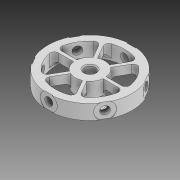
# Autodesk Inventor part: DrivePulley
Saved by Autodesk Inventor 2020 (Build 240168000, 168)
## iProperties
Created: 2021-05-16
Part Number: DrivePulley
Material: Generic
Document SubType Name: Modeling
Designer: DDeGo
Density: 1 g/cm^3
Appearance: Default
Author: DDeGo
Autodesk Inventor part; units mm, degrees
ref_plane "YZ Plane" through (0, 0, 0) normal (1, 0, 0) x (0, 1, 0)
ref_plane "XZ Plane" through (0, 0, 0) normal (0, 1, 0) x (-1, 0, 0)
sketch "Sketch1" plane through (0, 0, 0) normal (0, 0, 1) x (1, 0, 0)
  line L0 (5.5, 9.1) -> (5.5, 7.6)
  line L1 (5.5, 7.6) -> (4, 7.1)
  line L2 (4, 7.1) -> (4, 3.5)
  line L3 (4, 3.5) -> (5.5, 3)
  line L4 (5.5, 3) -> (5.5, 0)
  line L5 (5.5, 0) -> (2.57, 0)
  line L6 (2.57, 0) -> (2.57, 9.1)
  line L7 (2.57, 9.1) -> (5.5, 9.1)
  line L8 (2.57, 0) -> (0, 0) construction
  line L9 (0, 0) -> (0, 9.1) construction
  line L10 (0, 9.1) -> (2.57, 9.1) construction
  dimension "d1" = 3.6
  dimension "d2" = 1.5
  dimension "d3" = 3
  dimension "d4" = 0.5
  dimension "d5" = 1.5
  dimension "d15" = 2.57
  dimension "d16" = 4
  constraints: 22 end point, 4 perpendicular, 2 point on line, 1 equal length, 1 horizontal, 1 parallel, 1 vertical, 1 other
  measures "d1" distance of L2.start L3.start
  measures "d2" distance of L0.start L1.start
  measures "d3" distance of L4.start L4.end
  measures "d4" vertical distance of L3.start L4.start
  measures "d5" distance between parallel lines of L2 L4
  measures "d15" distance between parallel lines of L6 L9
  measures "d16" distance between parallel lines of L9 L2
revolve "Revolution1" add sketch "Sketch1" angle 360 about axis through (0, 0, 0) along (0, 1, 0)
sketch "Sketch2" plane through (0, 0, 0) normal (1, 0, 0) x (0, 1, 0)
  line L0 (9.1, 5.5) -> (9.1, -5.5) projected
  line L1 (9.1, 2.57) -> (9.1, -2.57) projected
  line L2 (9.1, -2.57) -> (17.1, -2.57)
  line L3 (17.1, -2.57) -> (17.1, -7)
  line L4 (17.1, -20) -> (10.1, -20)
  line L5 (10.1, -20) -> (10.1, -16.5)
  line L6 (10.1, -6.5) -> (9.1, -5.5)
  line L7 (9.1, 0) -> (17.1054, 0) construction
  line L8 (17.1, -16.5) -> (10.1, -16.5)
  line L9 (17.1, -7) -> (10.1, -7)
  line L10 (17.1, -7) -> (17.1, -16.5) construction
  line L11 (17.1, -16.5) -> (17.1, -20)
  line L12 (10.1, -16.5) -> (10.1, -7) construction
  line L13 (10.1, -7) -> (10.1, -6.5)
  point P0 (0, 0)
  dimension "d18" = 7
  dimension "d19" = 20
  dimension "d20" = 1
  dimension "d21" = 135
  dimension "d24" = 3.5
  dimension "d48" = 0.5
  constraints: 24 end point, 15 perpendicular, 2 horizontal, 2 point on line, 1 midpoint
  measures "d18" distance between parallel lines of L3 L5
  measures "d19" distance between parallel lines of L4 L7
  measures "d20" distance between parallel lines of L0 L5
  measures "d21" angle of L0 L6
  measures "d24" distance between parallel lines of L4 L8
  measures "d48" distance of L9.end L6.start
revolve "Revolution2" add sketch "Sketch2" angle 360 about axis through (0, 9.1, 0) along (0, 1, 0)
sketch "Sketch3" plane through (0, 17.1, 0) normal (0, 1, 0) x (1, 0, 0)
  line L0 (-4, 0.75) -> (-18, 0.75)
  line L1 (-18, 0.75) -> (-18, -0.75)
  line L2 (-18, -0.75) -> (-4, -0.75)
  line L3 (-4, -0.75) -> (-4, 0.75)
  line L4 (-4, 0.75) -> (-18, -0.75) construction
  line L5 (-18, 0.75) -> (-4, -0.75) construction
  line L6 (0, 0) -> (-11, 0) construction
  dimension "d25" = 11
  dimension "d26" = 14
  dimension "d27" = 1.5
  constraints: 14 end point, 2 horizontal, 2 midpoint, 2 parallel, 1 perpendicular
  measures "d25" distance of L6.start L6.end
  measures "d26" distance of L0.start L0.end
  measures "d27" distance of L0.end L1.end
extrude "Extrusion1" add sketch "Sketch3" against normal blind 4
pattern_circular "Circular Pattern1" count 6 over 360 about axis through (0, 13.6, 0) along (0, -1, 0) of "Extrusion1"
ref_plane "Work Plane1" through (0, 0, 11.5) normal (0, 0, 1) x (1, 0, 0)
sketch "Sketch4" plane through (0, 0, 11.5) normal (0, 0, 1) x (1, 0, 0)
  line L0 (-20, 10.1) -> (20, 10.1) construction
  line L1 (-20, 17.1) -> (20, 17.1) construction
  line L2 (0, 17.1) -> (0, 10.1) construction
  circle A0 centre (0, 13.6) radius 1.9
  point P0 (0, 0)
  dimension "d34" = 3.8
  constraints: 3 midpoint, 2 end point, 1 centre point
  measures "d34" diameter of A0
extrude "Extrusion2" cut sketch "Sketch4" along normal through all
ref_plane "Work Plane2" through (0, 13.6, 20) normal (0, 0, 1) x (1, 0, 0)
sketch "Sketch5" plane through (0, 13.6, 20) normal (0, 0, 1) x (1, 0, 0)
  spline S0 degree 8 poles (1.9, 0) (1.9, 0.1657) (1.8835, 0.3313) (1.8505, 0.4958) (1.8008, 0.6582) (1.734, 0.8172) (1.6495, 0.9713) (1.5468, 1.1185) (1.329, 1.3656) (1.2201, 1.4699) (1.0986, 1.567) (0.9648, 1.6549) (0.8196, 1.7313) (0.6639, 1.7942) (0.499, 1.8416) (0.1415, 1.904) (-0.0486, 1.9156) (-0.2394, 1.9053) (-0.4268, 1.8731) (-0.6067, 1.8205) (-0.7753, 1.75) (-0.9298, 1.6654) (-1.2829, 1.4254) (-1.4642, 1.253) (-1.6123, 1.0628) (-1.7287, 0.8604) (-1.8146, 0.6501) (-1.8715, 0.435) (-1.9, 0.2176) (-1.9, -0.1657) (-1.8835, -0.3313) (-1.8505, -0.4958) (-1.8008, -0.6582) (-1.734, -0.8172) (-1.6495, -0.9713) (-1.5468, -1.1185) (-1.3074, -1.3901) (-1.1692, -1.518) (-1.0111, -1.6345) (-0.8343, -1.7349) (-0.6412, -1.8149) (-0.4352, -1.8709) (-0.22, -1.9) (0.2015, -1.9) (0.3995, -1.8756) (0.5903, -1.8282) (0.7708, -1.7601) (0.9382, -1.6739) (1.0903, -1.5731) (1.2255, -1.4615) (1.4864, -1.2006) (1.607, -1.0452) (1.706, -0.8809) (1.7842, -0.7103) (1.8422, -0.5355) (1.8807, -0.3579) (1.9, -0.179) (1.9, 0) knots 0 0 0 0 0 0 0 0 0 0.126174 0.126174 0.126174 0.126174 0.126174 0.126174 0.126174 0.226013 0.226013 0.226013 0.226013 0.226013 0.226013 0.226013 0.333304 0.333304 0.333304 0.333304 0.333304 0.333304 0.333304 0.500214 0.500214 0.500214 0.500214 0.500214 0.500214 0.500214 0.627329 0.627329 0.627329 0.627329 0.627329 0.627329 0.627329 0.750487 0.750487 0.750487 0.750487 0.750487 0.750487 0.750487 0.863304 0.863304 0.863304 0.863304 0.863304 0.863304 0.863304 1 1 1 1 1 1 1 1 1 projected
  line L0 (-1.9, 0) -> (0, 0) construction
  line L1 (0, 0) -> (0, -1.9) construction
  circle A0 centre (0, 0) radius 4
  point P0 (0, -13.6)
  dimension "d37" = 8
  constraints: 4 end point, 1 centre point, 1 coincident, 1 horizontal, 1 perpendicular, 1 point on line, 2 other
  measures "d37" diameter of A0
extrude "Extrusion3" cut sketch "Sketch5" against normal blind 0.4
pattern_circular "Circular Pattern2" count 6 over 360 about axis through (0, 4.55, 0) along (0, -1, 0) of "Extrusion3", "Extrusion2"
fillet "Fillet1" radius 2 12 edges at (-7.592, 15.1, 14.6496) (-8.891, 15.1, 13.8996) (-16.4829, 15.1, 0.75) (-16.4829, 15.1, -0.75) (8.891, 15.1, 13.8996) (7.592, 15.1, 14.6496) (16.4829, 15.1, -0.75) (16.4829, 15.1, 0.75) (7.592, 15.1, -14.6496) (8.891, 15.1, -13.8996) (-7.592, 15.1, -14.6496) (-8.891, 15.1, -13.8996)
fillet "Fillet1" radius 2 12 edges at (16.5, 13.1, 0) (8.25, 13.1, -14.2894) (-8.25, 13.1, -14.2894) (-16.5, 13.1, 0) (-8.25, 13.1, 14.2894) (8.25, 13.1, 14.2894) (3.5, 13.1, 6.0622) (-3.5, 13.1, 6.0622) (7, 13.1, 0) (3.5, 13.1, -6.0622) (-3.5, 13.1, -6.0622) (-7, 13.1, 0)
chamfer "Chamfer1" distance 0.5 angle 45 2 edges at (0, 17.1, 2.57) (-2.57, 0, 0)
body "Solid1"
